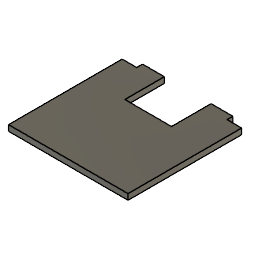
ultra achter (Autodesk Fusion 360 design; units mm, degrees)
part number: 2026-03-26-09-04-28-193
Autodesk Fusion 360 part; units mm, degrees
sketch "Sketch1" plane through (0, 0, 0) normal (0, 0, 1) x (1, 0, 0)
  line L0 (45.0489, 45.9669) -> (45.0489, -32.0331)
  line L1 (45.0489, -32.0331) -> (-36.9511, -32.0331)
  line L2 (-36.9511, -32.0331) -> (-36.9511, 45.9669)
  line L3 (-11.9511, 49.9669) -> (-11.9511, 32.8404)
  line L4 (-26.9511, 45.9669) -> (-26.9511, 49.9669)
  line L5 (35.0489, 49.9669) -> (35.0489, 45.9669)
  line L6 (20.0489, 32.8404) -> (20.0489, 49.9669)
  line L7 (-26.9511, 49.9669) -> (-11.9511, 49.9669)
  line L8 (-26.9511, 45.9669) -> (-36.9511, 45.9669)
  line L9 (-11.9511, 32.8404) -> (-10.4667, 32.8404)
  line L10 (-10.4667, 32.8404) -> (20.0489, 32.8404)
  line L11 (20.0489, 49.9669) -> (35.0489, 49.9669)
  line L12 (35.0489, 45.9669) -> (45.0489, 45.9669)
  constraint vertical L0
  constraint vertical L2
  constraint vertical L3
  constraint vertical L4
  constraint vertical L5
  constraint vertical L6
  constraint coincident L2 L8.end
  constraint perpendicular L2 L8
  constraint perpendicular L6 L10
  constraint perpendicular L5 L11
  constraint coincident L0 L12.end
  constraint perpendicular L0 L12
extrude "Extrude1" add sketch "Sketch1" along normal blind 4
extrude "Extrude2" cut 2 faces at (-11.4563, 32.8404, 1.3333) (-0.2948, 32.8404, 2.6667) along direction (0, -1, 0) blind 10
